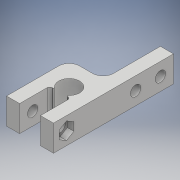
# Autodesk Inventor part: Camera_Bed_Detector
Saved by Autodesk Inventor 2017 (Build 210142000, 142)
## iProperties
Created: 2016-12-17
Part Number: Camera_Bed_Detector
Material: Generic
Document SubType Name: Modeling
Designer: willt
Density: 1 g/cm^3
Appearance: Default
Author: willt
Autodesk Inventor part; units mm, degrees
ref_plane "YZ Plane" through (0, 0, 0) normal (1, 0, 0) x (0, 1, 0)
ref_plane "XZ Plane" through (0, 0, 0) normal (0, 1, 0) x (-1, 0, 0)
ref_plane "XY Plane" through (0, 0, 0) normal (0, 0, 1) x (1, 0, 0)
sketch "Sketch1" plane through (0, 0, 0) normal (0, 1, 0) x (-1, 0, 0)
  line L0 (0, 2) -> (5, 2)
  line L1 (5, 2) -> (5, -16)
  line L2 (0, -20) -> (0, 2)
  line L3 (0, -44) -> (5, -44)
  line L4 (5, -44) -> (5, -33.4641)
  arc A0 (13, -29) -> (5, -29) centre (9, -29) ccw
  line L5 (9, -20) -> (14, -20)
  line L6 (18, -44) -> (13, -44)
  line L7 (13, -44) -> (13, -33.4641)
  line L8 (18, -24) -> (18, -44)
  line L9 (0, -20) -> (0, -44)
  arc A1 (5, -16) -> (9, -20) centre (9, -16) ccw
  arc A2 (18, -24) -> (14, -20) centre (14, -24) ccw
  circle A3 centre (9, -29) radius 4 construction
  line L10 (6, -32.4641) -> (6.2193, -32.4641)
  line L11 (12, -32.4641) -> (11.7807, -32.4641)
  arc A4 (5, -29) -> (6.3829, -32.025) centre (9, -29) ccw
  arc A5 (11.6171, -32.025) -> (13, -29) centre (9, -29) ccw
  arc A6 (6.2193, -32.4641) -> (6.3829, -32.025) centre (6.2193, -32.2141) ccw
  arc A7 (11.6171, -32.025) -> (11.7807, -32.4641) centre (11.7807, -32.2141) ccw
  arc A8 (6, -32.4641) -> (5, -33.4641) centre (6, -33.4641) ccw
  arc A9 (13, -33.4641) -> (12, -32.4641) centre (12, -33.4641) ccw
  point P0 (0, 0)
  point P1 (7, -32.4641)
  point P2 (11, -32.4641)
  dimension "d45" = 1
  constraints: 24 end point, 20 point on circle, 12 tangent, 9 centre point, 5 horizontal, 3 equal radius, 3 perpendicular, 3 point on line, 2 parallel, 1 coincident, 1 horizontal alignment, 3 other
  measures "d45" radius of A8
extrude "Extrusion1" add sketch "Sketch1" along normal blind 10
move or copy body "Move Body1" bodies to move or copy 1 copy no rotation origin (0, 0, 0) rotation axis (1, 0, 0) rotation angle -90 translate (0, 54, -34)
sketch "Sketch4" plane through (0, 10, -34) normal (1, 0, 0) x (0, 0, -1)
  line L0 (0, 46) -> (10, 46) construction
  line L1 (5, 46) -> (5, 41) construction
  circle A0 centre (5, 41) radius 2
  circle A1 centre (5, 31.5) radius 2
  circle A2 centre (5, 5) radius 2
  dimension "d29" = 5
  dimension "d30" = 4
  dimension "d31" = 4
  dimension "d32" = 4
  constraints: 3 centre point, 3 coincident, 2 end point, 1 midpoint, 1 vertical
  measures "d29" distance of L1.start L1.end
  measures "d30" diameter of A0
  measures "d31" diameter of A1
  measures "d32" diameter of A2
extrude "Extrusion3" cut sketch "Sketch4" against normal blind 5
sketch "Sketch5" plane through (0, 10, -34) normal (1, 0, 0) x (0, 0, -1)
  circle A0 centre (5, 5) radius 2 construction
  circle A1 centre (5, 5) radius 3.25 construction
  line L0 (8.25, 5) -> (6.625, 2.1854)
  line L1 (6.625, 2.1854) -> (3.375, 2.1854)
  line L2 (3.375, 2.1854) -> (1.75, 5)
  line L3 (1.75, 5) -> (3.375, 7.8146)
  line L4 (3.375, 7.8146) -> (6.625, 7.8146)
  line L5 (6.625, 7.8146) -> (8.25, 5)
  point P0 (-34, -10)
  dimension "d35" = 6.5
  constraints: 12 end point, 2 coincident, 1 horizontal alignment, 15 other
extrude "Extrusion4" cut sketch "Sketch5" against normal blind 2.5
sketch "Sketch6" plane through (-18, 10, -34) normal (-1, 0, 0) x (0, 0, 1)
  line L0 (0, 0) -> (-10, 0) construction
  line L1 (-5, 0) -> (-5, 5) construction
  circle A0 centre (-5, 5) radius 2
  point P0 (34, -10)
  dimension "d38" = 5
  dimension "d39" = 4
  constraints: 2 end point, 1 centre point, 1 coincident, 1 midpoint, 1 vertical
  measures "d38" distance of L1.start L1.end
  measures "d39" diameter of A0
extrude "Extrusion5" cut sketch "Sketch6" against normal blind 5
body "Solid1"
